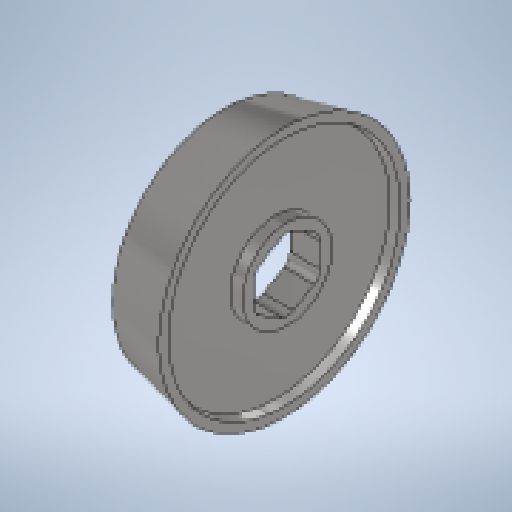
# Autodesk Inventor part: Clutch
Saved by Autodesk Inventor 2023.2 (Build 272271000, 271)
## iProperties
Created: 2024-01-10
Part Number: Clutch
Material: Stainless Steel
Document SubType Name: Modeling
Designer: Nathan Cai
Mass: 44.0483 g
Surface Area: 45.7106 cm^2
Volume: 5.50604 cm^3
Density: 8 g/cm^3
Appearance: Semi-Polished
Author: Nathan Cai
Autodesk Inventor part; units mm, degrees
ref_plane "YZ Plane" through (0, 0, 0) normal (1, 0, 0) x (0, 1, 0)
ref_plane "XZ Plane" through (0, 0, 0) normal (0, 1, 0) x (-1, 0, 0)
ref_plane "XY Plane" through (0, 0, 0) normal (0, 0, 1) x (1, 0, 0)
sketch "Sketch1" plane through (0, 0, 0) normal (0, 1, 0) x (-1, 0, 0)
  line L0 (0, 0) -> (3, 0) construction
  line L1 (3, 0) -> (3, -5.875) construction
  line L2 (3, -5.875) -> (0, -5.875) construction
  line L3 (0, -5.875) -> (0, 0) construction
  line L4 (0, -5.875) -> (3, -5.875)
  line L5 (3, -5.875) -> (3, -23)
  line L6 (3, -23) -> (0, -23)
  line L7 (0, -23) -> (0, -5.875)
  line L8 (8.5, -23) -> (-1.5, -23) construction
  line L9 (-1.5, -23) -> (-1.5, -17)
  line L10 (-1.5, -17) -> (8.5, -17)
  line L11 (8.5, -17) -> (8.5, -23)
  line L12 (-1.5, -21) -> (8.5, -18.7831)
  line L13 (-1.5, -19.4636) -> (8.5, -17.2466)
  line L14 (3, -5.875) -> (5, -5.875)
  line L15 (5, -5.875) -> (5, -9.875)
  line L16 (5, -9.875) -> (3, -9.875)
  line L17 (3, -9.875) -> (3, -5.875)
  line L18 (0, -5.875) -> (-2, -5.875)
  line L19 (-2, -5.875) -> (-2, -7.875)
  line L20 (-2, -7.875) -> (0, -7.875)
  line L21 (0, -7.875) -> (0, -5.875)
  point P0 (3, -17)
  point P1 (0, -17)
  point P2 (0, -19.131)
  point P3 (3, -18.466)
  point P4 (3, -9.875)
  point P5 (0, -7.875)
  dimension "d21" = 3
  dimension "d22" = 5.875
  dimension "d24" = 1.5
  dimension "d25" = 10
  dimension "d26" = 6
  dimension "d27" = 2
  dimension "d29" = 21
  dimension "d30" = 1.5
  dimension "d34" = 2
  dimension "d35" = 4
  dimension "d36" = 2
  dimension "d37" = 2
  dimension "d38" = 12.5
  constraints: 44 end point, 11 parallel, 6 point on line, 5 horizontal, 5 perpendicular
  measures "d21" distance of L1.end L2.end
  measures "d22" distance of L0.end L1.end
  measures "d24" distance between parallel lines of L7 L9
  measures "d25" distance between parallel lines of L9 L11
  measures "d26" distance between parallel lines of L8 L10
  measures "d27" distance from line of L8 L12.start
  measures "d29" distance from line of L0 L12.start
  measures "d30" distance between parallel lines of L12 L13
  measures "d34" distance of L15.end L16.end
  measures "d35" distance of L14.end L15.end
  measures "d36" distance of L20.end L19.end
  measures "d37" distance of L19.end L18.end
  measures "d38" angle of L8 L12
revolve "Revolution1" add sketch "Sketch1" angle 360 about axis through (0, 0, 0) along (-1, 0, 0) contours L4 L5 L10 L7 | L7 L20 L19 L18 | L10 L5 L13 L7 | L10 L11 L13 L5 | L13 L5 L12 L7 | L7 L12 L9 L13 | L13 L11 L12 L5
sketch "Sketch5" plane through (-3, 0, 0) normal (-1, 0, 0) x (0, 0, 1)
  line L0 (0, 0) -> (-5.875, 0) construction
  line L1 (-5.875, 3.3919) -> (0, 6.7839)
  line L2 (0, 6.7839) -> (5.875, 3.3919)
  line L3 (5.875, 3.3919) -> (5.875, -3.3919)
  line L4 (5.875, -3.3919) -> (0, -6.7839)
  line L5 (0, -6.7839) -> (-5.875, -3.3919)
  line L6 (-5.875, -3.3919) -> (-5.875, 3.3919)
  circle A0 centre (0, 0) radius 5.875 projected
  circle A1 centre (0, 0) radius 17 projected
  circle A2 centre (0, 0) radius 5.875 projected
  constraints: 14 end point, 2 coincident, 1 horizontal, 1 midpoint, 1 tangent, 13 other
extrude "Extrusion4" cut sketch "Sketch5" along normal through all both and the other way through all contours L1 A0 L6 | L1 L2 A0 | A0 | A0 L5 L6 | L2 L3 A0 | A0 L4 L5 | L3 L4 A0
fillet "Fillet4" radius 2 6 edges at (-0.5, -3.3919, -5.875) (-0.5, 3.3919, -5.875) (-0.5, 6.7839, 0) (-0.5, -6.7839, 0) (-0.5, -3.3919, 5.875) (-0.5, 3.3919, 5.875)
body "Solid1"
